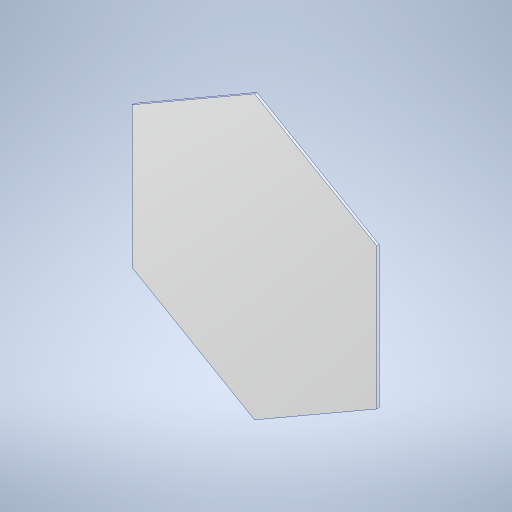
# Autodesk Inventor part: Bottom plate 2.5mm
Saved by Autodesk Inventor 2023 (Build 270158000, 158)
## iProperties
Created: 2022-06-23
Part Number: Bottom plate 2.5mm
Material: Aluminum 6061
Document SubType Name: Sheet Metal
Designer: earls
Density: 2.7 g/cm^3
Appearance: Aluminum - Flat
Sheet Metal Rule: Default
Author: earls
Autodesk Inventor part; units mm, degrees
ref_plane "YZ Plane" through (0, 0, 0) normal (1, 0, 0) x (0, 1, 0)
ref_plane "XZ Plane" through (0, 0, 0) normal (0, 1, 0) x (-1, 0, 0)
ref_plane "XY Plane" through (0, 0, 0) normal (0, 0, 1) x (1, 0, 0)
sketch "Sketch1" plane through (0, 0, 0) normal (0, 0, 1) x (1, 0, 0)
  line L0 (0, 150) -> (129.9038, 75)
  line L1 (129.9038, 75) -> (129.9038, -75)
  line L2 (129.9038, -75) -> (0, -150)
  line L3 (0, -150) -> (-129.9038, -75)
  line L4 (-129.9038, -75) -> (-129.9038, 75)
  line L5 (-129.9038, 75) -> (0, 150)
  point P0 (0, 0)
  point P1 (0, 0)
  dimension "d0" = 150
  constraints: 12 end point, 1 coincident, 13 other
  measures "d0" distance of L3.end L4.end
extrude "Extrusion1" add sketch "Sketch1" along normal blind 2.5
sketch "Sketch2" plane through (0, 0, 2.5) normal (0, 0, 1) x (1, 0, 0)
  circle A0 centre (0, 0) radius 5
  dimension "d3" = 10
  constraints: 1 centre point, 1 coincident
  measures "d3" diameter of A0
extrude "Extrusion2" cut sketch "Sketch2" against normal blind 10
sketch "Sketch3" plane through (0, 0, 2.5) normal (0, 0, 1) x (1, 0, 0)
  circle A0 centre (0, 0) radius 5
sheet face with bend "Face1" sketch "Sketch3" thickness 3.048 toward (0, 0, -1) bend radius 3.048
bend "Bend1"
equation "\"d6\" = Thickness"
equation "\"d7\" = BendRadius"
equation "\"d8\" = BendReliefWidth"
equation "\"d10\" = MinimumRemnant"
equation "\"d9\" = BendReliefDepth"
equation "\"d11\" = TransitionRadius"
equation "\"BendRadius\" = Thickness"
equation "\"BendReliefWidth\" = Thickness"
equation "\"BendReliefDepth\" = 0.5 * Thickness"
equation "\"CornerReliefSize\" = 4 * Thickness"
equation "\"MinimumRemnant\" = 2 * Thickness"
equation "\"TransitionRadius\" = BendRadius"
equation "\"JacobiRadiusSize\" = BendRadius"
equation "\"GapSize\" = Thickness"
equation "\"Thickness\" = 3.048"
body "Solid1"
